Autodesk Inventor part; units mm, degrees
(part 2 of 2)
sketch "Sketch19" plane through (0, 0, 0.5) normal (0, 0, 1) x (1, 0, 0)
  circle A0 centre (5.5, -12.3356) radius 0.0625 projected
  line L0 (5.5548, -12.3056) -> (5.7, -12.3056)
  line L1 (5.5548, -12.3656) -> (5.7, -12.3656)
  line L2 (5.7, -12.2156) -> (5.7, -12.3056)
  line L3 (5.71, -12.2056) -> (5.79, -12.2056)
  line L4 (5.8, -12.2156) -> (5.8, -12.2256)
  arc A1 (5.71, -12.2056) -> (5.7, -12.2156) centre (5.71, -12.2156) ccw
  arc A2 (5.8, -12.2156) -> (5.79, -12.2056) centre (5.79, -12.2156) ccw
  line L5 (5.7, -12.4556) -> (5.7, -12.3656)
  line L6 (5.71, -12.4656) -> (5.79, -12.4656)
  line L7 (5.8, -12.4556) -> (5.8, -12.4456)
  arc A3 (5.7, -12.4556) -> (5.71, -12.4656) centre (5.71, -12.4556) ccw
  arc A4 (5.79, -12.4656) -> (5.8, -12.4556) centre (5.79, -12.4556) ccw
  circle A5 centre (7.5, -12.3356) radius 0.0625 projected
  line L8 (7.4452, -12.3056) -> (7.3, -12.3056)
  line L9 (7.4452, -12.3656) -> (7.3, -12.3656)
  line L10 (7.3, -12.2156) -> (7.3, -12.3056)
  line L11 (7.29, -12.2056) -> (7.21, -12.2056)
  line L12 (7.2, -12.2156) -> (7.2, -12.2256)
  arc A6 (7.3, -12.2156) -> (7.29, -12.2056) centre (7.29, -12.2156) ccw
  arc A7 (7.21, -12.2056) -> (7.2, -12.2156) centre (7.21, -12.2156) ccw
  arc A8 (7.29, -12.4656) -> (7.3, -12.4556) centre (7.29, -12.4556) ccw
  line L13 (7.3, -12.4556) -> (7.3, -12.3656)
  line L14 (7.29, -12.4656) -> (7.21, -12.4656)
  arc A9 (7.2, -12.4556) -> (7.21, -12.4656) centre (7.21, -12.4556) ccw
  line L15 (7.2, -12.4556) -> (7.2, -12.4456)
  line L16 (5.8, -12.4456) -> (7.2, -12.4456)
  line L17 (5.8, -12.2256) -> (7.2, -12.2256)
  line L18 (5.5548, -10.3056) -> (5.7, -10.3056)
  line L19 (5.5548, -10.3656) -> (5.7, -10.3656)
  line L20 (5.7, -10.2156) -> (5.7, -10.3056)
  line L21 (5.71, -10.2056) -> (5.79, -10.2056)
  line L22 (5.8, -10.2156) -> (5.8, -10.2256)
  arc A10 (5.71, -10.2056) -> (5.7, -10.2156) centre (5.71, -10.2156) ccw
  arc A11 (5.8, -10.2156) -> (5.79, -10.2056) centre (5.79, -10.2156) ccw
  arc A12 (5.7, -10.4556) -> (5.71, -10.4656) centre (5.71, -10.4556) ccw
  line L23 (5.7, -10.4556) -> (5.7, -10.3656)
  line L24 (5.71, -10.4656) -> (5.79, -10.4656)
  arc A13 (5.79, -10.4656) -> (5.8, -10.4556) centre (5.79, -10.4556) ccw
  line L25 (5.8, -10.4556) -> (5.8, -10.4456)
  line L26 (7.4452, -10.3056) -> (7.3, -10.3056)
  line L27 (7.4452, -10.3656) -> (7.3, -10.3656)
  line L28 (7.3, -10.4556) -> (7.3, -10.3656)
  arc A14 (7.29, -10.4656) -> (7.3, -10.4556) centre (7.29, -10.4556) ccw
  line L29 (7.29, -10.4656) -> (7.21, -10.4656)
  arc A15 (7.2, -10.4556) -> (7.21, -10.4656) centre (7.21, -10.4556) ccw
  line L30 (7.2, -10.2156) -> (7.2, -10.2256)
  line L31 (7.29, -10.2056) -> (7.21, -10.2056)
  line L32 (7.3, -10.2156) -> (7.3, -10.3056)
  arc A16 (7.3, -10.2156) -> (7.29, -10.2056) centre (7.29, -10.2156) ccw
  arc A17 (7.21, -10.2056) -> (7.2, -10.2156) centre (7.21, -10.2156) ccw
  line L33 (7.2, -10.4556) -> (7.2, -10.4456)
  line L34 (5.8, -10.4456) -> (7.2, -10.4456)
  line L35 (5.8, -10.2256) -> (7.2, -10.2256)
  line L36 (5.5548, -9.6806) -> (5.7, -9.6806)
  line L37 (5.5548, -9.7406) -> (5.7, -9.7406)
  line L38 (5.7, -9.5906) -> (5.7, -9.6806)
  line L39 (5.71, -9.5806) -> (5.79, -9.5806)
  line L40 (5.8, -9.5906) -> (5.8, -9.6006)
  arc A18 (5.71, -9.5806) -> (5.7, -9.5906) centre (5.71, -9.5906) ccw
  arc A19 (5.8, -9.5906) -> (5.79, -9.5806) centre (5.79, -9.5906) ccw
  arc A20 (5.7, -9.8306) -> (5.71, -9.8406) centre (5.71, -9.8306) ccw
  line L41 (5.7, -9.8306) -> (5.7, -9.7406)
  line L42 (5.71, -9.8406) -> (5.79, -9.8406)
  arc A21 (5.79, -9.8406) -> (5.8, -9.8306) centre (5.79, -9.8306) ccw
  line L43 (5.8, -9.8306) -> (5.8, -9.8206)
  line L44 (7.4452, -9.6806) -> (7.3, -9.6806)
  line L45 (7.4452, -9.7406) -> (7.3, -9.7406)
  line L46 (7.3, -9.8306) -> (7.3, -9.7406)
  arc A22 (7.29, -9.8406) -> (7.3, -9.8306) centre (7.29, -9.8306) ccw
  line L47 (7.29, -9.8406) -> (7.21, -9.8406)
  arc A23 (7.2, -9.8306) -> (7.21, -9.8406) centre (7.21, -9.8306) ccw
  line L48 (7.2, -9.5906) -> (7.2, -9.6006)
  line L49 (7.29, -9.5806) -> (7.21, -9.5806)
  line L50 (7.3, -9.5906) -> (7.3, -9.6806)
  arc A24 (7.3, -9.5906) -> (7.29, -9.5806) centre (7.29, -9.5906) ccw
  arc A25 (7.21, -9.5806) -> (7.2, -9.5906) centre (7.21, -9.5906) ccw
  line L51 (7.2, -9.8306) -> (7.2, -9.8206)
  line L52 (5.8, -9.8206) -> (7.2, -9.8206)
  line L53 (5.8, -9.6006) -> (7.2, -9.6006)
  line L54 (5.5548, -9.0556) -> (5.7, -9.0556)
  line L55 (5.5548, -9.1156) -> (5.7, -9.1156)
  line L56 (5.7, -8.9656) -> (5.7, -9.0556)
  line L57 (5.71, -8.9556) -> (5.79, -8.9556)
  line L58 (5.8, -8.9656) -> (5.8, -8.9756)
  arc A26 (5.71, -8.9556) -> (5.7, -8.9656) centre (5.71, -8.9656) ccw
  arc A27 (5.8, -8.9656) -> (5.79, -8.9556) centre (5.79, -8.9656) ccw
  arc A28 (5.7, -9.2056) -> (5.71, -9.2156) centre (5.71, -9.2056) ccw
  line L59 (5.7, -9.2056) -> (5.7, -9.1156)
  line L60 (5.71, -9.2156) -> (5.79, -9.2156)
  arc A29 (5.79, -9.2156) -> (5.8, -9.2056) centre (5.79, -9.2056) ccw
  line L61 (5.8, -9.2056) -> (5.8, -9.1956)
  line L62 (7.4452, -9.0556) -> (7.3, -9.0556)
  line L63 (7.4452, -9.1156) -> (7.3, -9.1156)
  line L64 (7.3, -9.2056) -> (7.3, -9.1156)
  arc A30 (7.29, -9.2156) -> (7.3, -9.2056) centre (7.29, -9.2056) ccw
  line L65 (7.29, -9.2156) -> (7.21, -9.2156)
  arc A31 (7.2, -9.2056) -> (7.21, -9.2156) centre (7.21, -9.2056) ccw
  line L66 (7.2, -8.9656) -> (7.2, -8.9756)
  line L67 (7.29, -8.9556) -> (7.21, -8.9556)
  line L68 (7.3, -8.9656) -> (7.3, -9.0556)
  arc A32 (7.3, -8.9656) -> (7.29, -8.9556) centre (7.29, -8.9656) ccw
  arc A33 (7.21, -8.9556) -> (7.2, -8.9656) centre (7.21, -8.9656) ccw
  line L69 (7.2, -9.2056) -> (7.2, -9.1956)
  line L70 (5.8, -9.1956) -> (7.2, -9.1956)
  line L71 (5.8, -8.9756) -> (7.2, -8.9756)
  line L72 (5.5548, -8.4306) -> (5.7, -8.4306)
  line L73 (5.5548, -8.4906) -> (5.7, -8.4906)
  line L74 (5.7, -8.3406) -> (5.7, -8.4306)
  line L75 (5.71, -8.3306) -> (5.79, -8.3306)
  line L76 (5.8, -8.3406) -> (5.8, -8.3506)
  arc A34 (5.71, -8.3306) -> (5.7, -8.3406) centre (5.71, -8.3406) ccw
  arc A35 (5.8, -8.3406) -> (5.79, -8.3306) centre (5.79, -8.3406) ccw
  arc A36 (5.7, -8.5806) -> (5.71, -8.5906) centre (5.71, -8.5806) ccw
  line L77 (5.7, -8.5806) -> (5.7, -8.4906)
  line L78 (5.71, -8.5906) -> (5.79, -8.5906)
  arc A37 (5.79, -8.5906) -> (5.8, -8.5806) centre (5.79, -8.5806) ccw
  line L79 (5.8, -8.5806) -> (5.8, -8.5706)
  line L80 (7.4452, -8.4306) -> (7.3, -8.4306)
  line L81 (7.4452, -8.4906) -> (7.3, -8.4906)
  line L82 (7.3, -8.5806) -> (7.3, -8.4906)
  arc A38 (7.29, -8.5906) -> (7.3, -8.5806) centre (7.29, -8.5806) ccw
  line L83 (7.29, -8.5906) -> (7.21, -8.5906)
  arc A39 (7.2, -8.5806) -> (7.21, -8.5906) centre (7.21, -8.5806) ccw
  line L84 (7.2, -8.3406) -> (7.2, -8.3506)
  line L85 (7.29, -8.3306) -> (7.21, -8.3306)
  line L86 (7.3, -8.3406) -> (7.3, -8.4306)
  arc A40 (7.3, -8.3406) -> (7.29, -8.3306) centre (7.29, -8.3406) ccw
  arc A41 (7.21, -8.3306) -> (7.2, -8.3406) centre (7.21, -8.3406) ccw
  line L87 (7.2, -8.5806) -> (7.2, -8.5706)
  line L88 (5.8, -8.5706) -> (7.2, -8.5706)
  line L89 (5.8, -8.3506) -> (7.2, -8.3506)
  line L90 (5.5548, -7.8056) -> (5.7, -7.8056)
  line L91 (5.5548, -7.8656) -> (5.7, -7.8656)
  line L92 (5.7, -7.7156) -> (5.7, -7.8056)
  line L93 (5.71, -7.7056) -> (5.79, -7.7056)
  line L94 (5.8, -7.7156) -> (5.8, -7.7256)
  arc A42 (5.71, -7.7056) -> (5.7, -7.7156) centre (5.71, -7.7156) ccw
  arc A43 (5.8, -7.7156) -> (5.79, -7.7056) centre (5.79, -7.7156) ccw
  arc A44 (5.7, -7.9556) -> (5.71, -7.9656) centre (5.71, -7.9556) ccw
  line L95 (5.7, -7.9556) -> (5.7, -7.8656)
  line L96 (5.71, -7.9656) -> (5.79, -7.9656)
  arc A45 (5.79, -7.9656) -> (5.8, -7.9556) centre (5.79, -7.9556) ccw
  line L97 (5.8, -7.9556) -> (5.8, -7.9456)
  line L98 (7.4452, -7.8056) -> (7.3, -7.8056)
  line L99 (7.4452, -7.8656) -> (7.3, -7.8656)
  line L100 (7.3, -7.9556) -> (7.3, -7.8656)
  arc A46 (7.29, -7.9656) -> (7.3, -7.9556) centre (7.29, -7.9556) ccw
  line L101 (7.29, -7.9656) -> (7.21, -7.9656)
  arc A47 (7.2, -7.9556) -> (7.21, -7.9656) centre (7.21, -7.9556) ccw
  line L102 (7.2, -7.7156) -> (7.2, -7.7256)
  line L103 (7.29, -7.7056) -> (7.21, -7.7056)
  line L104 (7.3, -7.7156) -> (7.3, -7.8056)
  arc A48 (7.3, -7.7156) -> (7.29, -7.7056) centre (7.29, -7.7156) ccw
  arc A49 (7.21, -7.7056) -> (7.2, -7.7156) centre (7.21, -7.7156) ccw
  line L105 (7.2, -7.9556) -> (7.2, -7.9456)
  line L106 (5.8, -7.9456) -> (7.2, -7.9456)
  line L107 (5.8, -7.7256) -> (7.2, -7.7256)
  line L108 (5.5548, -7.1806) -> (5.7, -7.1806)
  line L109 (5.5548, -7.2406) -> (5.7, -7.2406)
  line L110 (5.7, -7.0906) -> (5.7, -7.1806)
  line L111 (5.71, -7.0806) -> (5.79, -7.0806)
  line L112 (5.8, -7.0906) -> (5.8, -7.1006)
  arc A50 (5.71, -7.0806) -> (5.7, -7.0906) centre (5.71, -7.0906) ccw
  arc A51 (5.8, -7.0906) -> (5.79, -7.0806) centre (5.79, -7.0906) ccw
  arc A52 (5.7, -7.3306) -> (5.71, -7.3406) centre (5.71, -7.3306) ccw
  line L113 (5.7, -7.3306) -> (5.7, -7.2406)
  line L114 (5.71, -7.3406) -> (5.79, -7.3406)
  arc A53 (5.79, -7.3406) -> (5.8, -7.3306) centre (5.79, -7.3306) ccw
  line L115 (5.8, -7.3306) -> (5.8, -7.3206)
  line L116 (7.4452, -7.1806) -> (7.3, -7.1806)
  line L117 (7.4452, -7.2406) -> (7.3, -7.2406)
  line L118 (7.3, -7.3306) -> (7.3, -7.2406)
  arc A54 (7.29, -7.3406) -> (7.3, -7.3306) centre (7.29, -7.3306) ccw
  line L119 (7.29, -7.3406) -> (7.21, -7.3406)
  arc A55 (7.2, -7.3306) -> (7.21, -7.3406) centre (7.21, -7.3306) ccw
  line L120 (7.2, -7.0906) -> (7.2, -7.1006)
  line L121 (7.29, -7.0806) -> (7.21, -7.0806)
  line L122 (7.3, -7.0906) -> (7.3, -7.1806)
  arc A56 (7.3, -7.0906) -> (7.29, -7.0806) centre (7.29, -7.0906) ccw
  arc A57 (7.21, -7.0806) -> (7.2, -7.0906) centre (7.21, -7.0906) ccw
  line L123 (7.2, -7.3306) -> (7.2, -7.3206)
  line L124 (5.8, -7.3206) -> (7.2, -7.3206)
  line L125 (5.8, -7.1006) -> (7.2, -7.1006)
  line L126 (5.5548, -6.6806) -> (5.7, -6.6806)
  line L127 (5.5548, -6.7406) -> (5.7, -6.7406)
  line L128 (5.7, -6.5906) -> (5.7, -6.6806)
  line L129 (5.71, -6.5806) -> (5.79, -6.5806)
  line L130 (5.8, -6.5906) -> (5.8, -6.6006)
  arc A58 (5.71, -6.5806) -> (5.7, -6.5906) centre (5.71, -6.5906) ccw
  arc A59 (5.8, -6.5906) -> (5.79, -6.5806) centre (5.79, -6.5906) ccw
  arc A60 (5.7, -6.8306) -> (5.71, -6.8406) centre (5.71, -6.8306) ccw
  line L131 (5.7, -6.8306) -> (5.7, -6.7406)
  line L132 (5.71, -6.8406) -> (5.79, -6.8406)
  arc A61 (5.79, -6.8406) -> (5.8, -6.8306) centre (5.79, -6.8306) ccw
  line L133 (5.8, -6.8306) -> (5.8, -6.8206)
  line L134 (7.4452, -6.6806) -> (7.3, -6.6806)
  line L135 (7.4452, -6.7406) -> (7.3, -6.7406)
  line L136 (7.3, -6.8306) -> (7.3, -6.7406)
  arc A62 (7.29, -6.8406) -> (7.3, -6.8306) centre (7.29, -6.8306) ccw
  line L137 (7.29, -6.8406) -> (7.21, -6.8406)
  arc A63 (7.2, -6.8306) -> (7.21, -6.8406) centre (7.21, -6.8306) ccw
  line L138 (7.2, -6.5906) -> (7.2, -6.6006)
  line L139 (7.29, -6.5806) -> (7.21, -6.5806)
  line L140 (7.3, -6.5906) -> (7.3, -6.6806)
  arc A64 (7.3, -6.5906) -> (7.29, -6.5806) centre (7.29, -6.5906) ccw
  arc A65 (7.21, -6.5806) -> (7.2, -6.5906) centre (7.21, -6.5906) ccw
  line L141 (7.2, -6.8306) -> (7.2, -6.8206)
  line L142 (5.8, -6.8206) -> (7.2, -6.8206)
  line L143 (5.8, -6.6006) -> (7.2, -6.6006)
  circle A66 centre (5.5, -7.8356) radius 0.0625 projected
  circle A67 centre (5.5, -7.8356) radius 0.0625
  circle A68 centre (5.5, -7.2106) radius 0.0625 projected
  circle A69 centre (5.5, -7.2106) radius 0.0625
  circle A70 centre (5.5, -6.7106) radius 0.0625 projected
  circle A71 centre (5.5, -6.7106) radius 0.0625
  circle A72 centre (7.5, -7.2106) radius 0.0625 projected
  circle A73 centre (7.5, -7.2106) radius 0.0625
  circle A74 centre (7.5, -6.7106) radius 0.0625 projected
  circle A75 centre (7.5, -6.7106) radius 0.0625
  circle A76 centre (7.5, -7.8356) radius 0.0625 projected
  circle A77 centre (7.5, -7.8356) radius 0.0625
  circle A78 centre (7.5, -8.4606) radius 0.0625 projected
  circle A79 centre (7.5, -8.4606) radius 0.0625
  circle A80 centre (7.5, -9.0856) radius 0.0625 projected
  circle A81 centre (7.5, -9.0856) radius 0.0625
  circle A82 centre (5.5, -9.0856) radius 0.0625 projected
  circle A83 centre (5.5, -9.0856) radius 0.0625
  circle A84 centre (5.5, -8.4606) radius 0.0625 projected
  circle A85 centre (5.5, -8.4606) radius 0.0625
  circle A86 centre (5.5, -10.3356) radius 0.0625 projected
  circle A87 centre (5.5, -10.3356) radius 0.0625
  circle A88 centre (5.5, -9.7106) radius 0.0625 projected
  circle A89 centre (5.5, -9.7106) radius 0.0625
  circle A90 centre (7.5, -9.7106) radius 0.0625 projected
  circle A91 centre (7.5, -9.7106) radius 0.0625
  circle A92 centre (7.5, -10.3356) radius 0.0625 projected
  circle A93 centre (7.5, -10.3356) radius 0.0625
  point P0 (0, 0)
  constraints: 288 end point, 132 point on circle, 64 centre point, 32 tangent, 24 horizontal, 14 coincident, 8 equal radius, 8 parallel, 8 vertical, 42 other
extrude "Extrusion11" cut sketch "Sketch19" against normal blind 0.001 contours A0 L0 L2 A1 L3 A2 L4 L17 L12 A7 L11 A6 L10 L8 A5 L9 L13 A8 L14 A9 L15 L16 L7 A4 L6 A3 L5 L1 | L18 L20 A10 L21 A11 L22 L35 L30 A17 L31 A16 L32 L26 A92 L27 L28 A14 L29 A15 L33 L34 L25 A13 L24 A12 L23 L19 A86 | L36 L38 A18 L39 A19 L40 L53 L48 A25 L49 A24 L50 L44 A90 L45 L46 A22 L47 A23 L51 L52 L43 A21 L42 A20 L41 L37 A88 | L54 L56 A26 L57 A27 L58 L71 L66 A33 L67 A32 L68 L62 A80 L63 L64 A30 L65 A31 L69 L70 L61 A29 L60 A28 L59 L55 A82 | L72 L74 A34 L75 A35 L76 L89 L84 A41 L85 A40 L86 L80 A78 L81 L82 A38 L83 A39 L87 L88 L79 A37 L78 A36 L77 L73 A84 | L90 L92 A42 L93 A43 L94 L107 L102 A49 L103 A48 L104 L98 A76 L99 L100 A46 L101 A47 L105 L106 L97 A45 L96 A44 L95 L91 A66 | L108 L110 A50 L111 A51 L112 L125 L120 A57 L121 A56 L122 L116 A72 L117 L118 A54 L119 A55 L123 L124 L115 A53 L114 A52 L113 L109 A68 | L126 L128 A58 L129 A59 L130 L143 L138 A65 L139 A64 L140 L134 A74 L135 L136 A62 L137 A63 L141 L142 L133 A61 L132 A60 L131 L127 A70
sketch "Sketch20" plane through (0, 0, 0.5) normal (0, 0, 1) x (1, 0, 0)
  line L0 (9.2529, -6.0349) -> (9.353, -6.0349) construction
  line L1 (9.353, -6.0349) -> (9.353, -6.1134) construction
  line L2 (9.353, -6.1134) -> (9.2529, -6.1134) construction
  line L3 (9.2529, -6.1134) -> (9.2529, -6.0349) construction
  point P0 (0, 0)
  constraints: 2 other
sketch "Sketch21" plane through (0, 0, 0.5) normal (0, 0, 1) x (1, 0, 0)
  line L0 (2.475, -6) -> (2.475, -5.85)
  line L1 (2.475, -5.85) -> (2.775, -5.85)
  line L2 (2.775, -5.85) -> (2.775, -12.35)
  line L3 (2.775, -12.35) -> (2.475, -12.35)
  line L4 (2.475, -12.35) -> (2.475, -6)
  line L5 (6.4126, -6.6715) -> (6.6377, -6.6715) construction
  line L6 (6.6377, -6.6715) -> (6.6377, -6.7316) construction
  line L7 (6.6377, -6.7316) -> (6.4126, -6.7316) construction
  line L8 (6.4126, -6.7316) -> (6.4126, -6.6715) construction
  line L9 (6.4225, -7.1608) -> (6.6476, -7.1608) construction
  line L10 (6.6476, -7.1608) -> (6.6476, -7.221) construction
  line L11 (6.6476, -7.221) -> (6.4225, -7.221) construction
  line L12 (6.4225, -7.221) -> (6.4225, -7.1608) construction
  line L13 (6.4217, -7.788) -> (6.6468, -7.788) construction
  line L14 (6.6468, -7.788) -> (6.6468, -7.8482) construction
  line L15 (6.6468, -7.8482) -> (6.4217, -7.8482) construction
  line L16 (6.4217, -7.8482) -> (6.4217, -7.788) construction
  line L17 (3.1, -6) -> (3.1, -5.85)
  line L18 (3.725, -6) -> (3.725, -5.85)
  line L19 (4.35, -6) -> (4.35, -5.85)
  line L20 (3.1, -5.85) -> (3.4, -5.85)
  line L21 (3.4, -5.85) -> (3.4, -12.35)
  line L22 (3.4, -12.35) -> (3.1, -12.35)
  line L23 (3.1, -12.35) -> (3.1, -6)
  line L24 (3.725, -5.85) -> (4.025, -5.85)
  line L25 (4.025, -5.85) -> (4.025, -12.35)
  line L26 (4.025, -12.35) -> (3.725, -12.35)
  line L27 (3.725, -12.35) -> (3.725, -6)
  line L28 (4.35, -5.85) -> (4.65, -5.85)
  line L29 (4.65, -5.85) -> (4.65, -12.35)
  line L30 (4.65, -12.35) -> (4.35, -12.35)
  line L31 (4.35, -12.35) -> (4.35, -6)
  line L32 (6.4642, -8.4748) -> (6.4642, -8.4147) construction
  line L33 (6.4642, -8.4147) -> (6.6262, -8.4147) construction
  line L34 (6.6262, -8.4147) -> (6.6262, -8.4748) construction
  line L35 (6.6262, -8.4748) -> (6.4642, -8.4748) construction
  line L36 (6.4337, -9.0961) -> (6.4337, -9.036) construction
  line L37 (6.4337, -9.036) -> (6.6588, -9.036) construction
  line L38 (6.6588, -9.036) -> (6.6588, -9.0961) construction
  line L39 (6.6588, -9.0961) -> (6.4337, -9.0961) construction
  line L40 (6.4323, -9.7147) -> (6.4323, -9.6546) construction
  line L41 (6.4323, -9.6546) -> (6.6574, -9.6546) construction
  line L42 (6.6574, -9.6546) -> (6.6574, -9.7147) construction
  line L43 (6.6574, -9.7147) -> (6.4323, -9.7147) construction
  line L44 (6.4255, -10.3617) -> (6.4255, -10.3016) construction
  line L45 (6.4255, -10.3016) -> (6.6506, -10.3016) construction
  line L46 (6.6506, -10.3016) -> (6.6506, -10.3617) construction
  line L47 (6.6506, -10.3617) -> (6.4255, -10.3617) construction
  line L48 (6.4342, -12.383) -> (6.4342, -12.2817) construction
  line L49 (6.4342, -12.2817) -> (6.6593, -12.2817) construction
  line L50 (6.6593, -12.2817) -> (6.6593, -12.383) construction
  line L51 (6.6593, -12.383) -> (6.4342, -12.383) construction
  line L52 (5, -7) -> (4.35, -7)
  line L53 (4.35, -8.6523) -> (5.1177, -8.6523)
  line L54 (5.1177, -8.6523) -> (5.1177, -7)
  line L55 (5, -7) -> (5.1177, -7)
  line L56 (9.39, -10.3668) -> (9.39, -8.5018)
  line L57 (8.79, -8.5018) -> (8.79, -10.3668)
  line L58 (8.79, -9.4343) -> (8.79, -9.2843)
  line L59 (8.79, -9.2843) -> (8.89, -9.2843)
  line L60 (8.89, -9.2843) -> (8.89, -9.5843)
  line L61 (8.89, -9.5843) -> (8.79, -9.5843)
  line L62 (9.69, -9.4343) -> (9.69, -9.1843)
  line L63 (9.69, -9.1843) -> (9.39, -9.1843)
  line L64 (9.69, -9.4343) -> (9.69, -9.6843)
  line L65 (9.69, -9.6843) -> (9.39, -9.6843)
  line L66 (8.79, -8.5018) -> (9.39, -8.5018)
  line L67 (8.79, -10.3668) -> (9.39, -10.3668)
  line L68 (9.29, -9.4343) -> (9.29, -9.0843)
  line L69 (9.29, -9.0843) -> (9.39, -9.0843)
  line L70 (9.29, -9.4343) -> (9.29, -9.7843)
  line L71 (9.29, -9.7843) -> (9.39, -9.7843)
  point P0 (0, 0)
  constraints: 80 end point, 13 perpendicular, 9 point on line, 6 vertical, 4 horizontal, 1 midpoint, 16 other
sketch "Sketch22" plane through (0, 0, 0) normal (0, 0, -1) x (-1, 0, 0)
  circle A0 centre (-9.0887, -11.003) radius 0.1 projected
  line L0 (-9.3887, -11.003) -> (-9.3887, -10.703)
  circle A1 centre (-8.6887, -11.003) radius 0.1 projected
  line L1 (-8.3887, -11.003) -> (-8.3887, -10.703)
  line L2 (-8.3887, -10.703) -> (-9.3887, -10.703)
  circle A2 centre (-8.8887, -12.3316) radius 0.1 projected
  line L3 (-9.3887, -11.003) -> (-9.3887, -12.6316)
  line L4 (-9.3887, -12.6316) -> (-8.3887, -12.6316)
  line L5 (-8.3887, -12.6316) -> (-8.3887, -11.003)
  circle A3 centre (-8.2121, -3.39) radius 0.1 projected
  line L6 (-7.9121, -3.39) -> (-7.9121, -3.69)
  circle A4 centre (-8.4104, -2.44) radius 0.1 projected
  line L7 (-8.4104, -2.14) -> (-7.9121, -2.14)
  circle A5 centre (-8.6121, -3.3893) radius 0.1 projected
  line L8 (-8.9121, -3.3893) -> (-8.9121, -3.6893)
  line L9 (-7.9121, -3.69) -> (-8.9121, -3.6893)
  line L10 (-8.9121, -3.3893) -> (-8.9121, -2.4893)
  line L11 (-8.9121, -2.4893) -> (-8.9121, -2.14)
  line L12 (-8.4104, -2.14) -> (-8.9121, -2.14)
  line L13 (-7.9121, -3.39) -> (-7.9121, -2.14)
  point P0 (0, 0)
  constraints: 28 end point, 4 vertical, 2 perpendicular, 1 horizontal
extrude "Extrusion12" add sketch "Sketch22" along normal blind 0.001
sketch "Sketch23" plane through (0, 0, 0.5) normal (0, 0, 1) x (1, 0, 0)
  line L0 (6.4364, -6.8881) -> (6.5968, -6.8881) construction
  line L1 (6.5968, -6.8881) -> (6.5968, -6.992) construction
  line L2 (6.5968, -6.992) -> (6.4364, -6.992) construction
  line L3 (6.4364, -6.992) -> (6.4364, -6.8881) construction
  line L4 (6.4361, -7.4082) -> (6.5965, -7.4082) construction
  line L5 (6.5965, -7.4082) -> (6.5965, -7.5082) construction
  line L6 (6.5965, -7.5082) -> (6.4361, -7.5082) construction
  line L7 (6.4361, -7.5082) -> (6.4361, -7.4082) construction
  line L8 (6.4442, -8.0322) -> (6.6046, -8.0322) construction
  line L9 (6.6046, -8.0322) -> (6.6046, -8.1367) construction
  line L10 (6.6046, -8.1367) -> (6.4442, -8.1367) construction
  line L11 (6.4442, -8.1367) -> (6.4442, -8.0322) construction
  line L12 (6.4449, -8.6472) -> (6.6053, -8.6472) construction
  line L13 (6.6053, -8.6472) -> (6.6053, -8.7472) construction
  line L14 (6.6053, -8.7472) -> (6.4449, -8.7472) construction
  line L15 (6.4449, -8.7472) -> (6.4449, -8.6472) construction
  line L16 (6.4675, -9.2967) -> (6.6278, -9.2967) construction
  line L17 (6.6278, -9.2967) -> (6.6278, -9.3971) construction
  line L18 (6.6278, -9.3971) -> (6.4675, -9.3971) construction
  line L19 (6.4675, -9.3971) -> (6.4675, -9.2967) construction
  line L20 (6.4727, -9.9151) -> (6.6331, -9.9151) construction
  line L21 (6.6331, -9.9151) -> (6.6331, -10.0172) construction
  line L22 (6.6331, -10.0172) -> (6.4727, -10.0172) construction
  line L23 (6.4727, -10.0172) -> (6.4727, -9.9151) construction
  line L24 (6.4883, -10.5491) -> (6.6486, -10.5491) construction
  line L25 (6.6486, -10.5491) -> (6.6486, -10.6512) construction
  line L26 (6.6486, -10.6512) -> (6.4883, -10.6512) construction
  line L27 (6.4883, -10.6512) -> (6.4883, -10.5491) construction
  line L28 (5.5344, -10.7366) -> (6.1019, -10.7366) construction
  line L29 (6.1019, -10.7366) -> (6.1019, -11.0038) construction
  line L30 (6.1019, -11.0038) -> (5.5344, -11.0038) construction
  line L31 (5.5344, -11.0038) -> (5.5344, -10.7366) construction
  line L32 (5.6586, -11.1538) -> (5.8162, -11.1538) construction
  line L33 (5.8162, -11.1538) -> (5.8162, -11.2574) construction
  line L34 (5.8162, -11.2574) -> (5.6586, -11.2574) construction
  line L35 (5.6586, -11.2574) -> (5.6586, -11.1538) construction
  line L36 (6.912, -11.1463) -> (7.0674, -11.1463) construction
  line L37 (7.0674, -11.1463) -> (7.0674, -11.2466) construction
  line L38 (7.0674, -11.2466) -> (6.912, -11.2466) construction
  line L39 (6.912, -11.2466) -> (6.912, -11.1463) construction
  line L40 (6.4628, -12.5696) -> (6.6231, -12.5696) construction
  line L41 (6.6231, -12.5696) -> (6.6231, -12.6738) construction
  line L42 (6.6231, -12.6738) -> (6.4628, -12.6738) construction
  line L43 (6.4628, -12.6738) -> (6.4628, -12.5696) construction
  point P0 (0, 0)
  constraints: 22 other
sketch "Sketch24" plane through (0, 0, 0.5) normal (0, 0, 1) x (1, 0, 0)
  circle A0 centre (7.1, -11.7731) radius 0.0625 projected
  circle A1 centre (7.1, -11.7731) radius 0.0625
  circle A2 centre (5.5, -11.7731) radius 0.0625
  point P0 (0, 0)
  dimension "d499" = 0.125
  constraints: 2 centre point, 1 coincident
  measures "d499" diameter of A2
extrude "Extrusion13" cut sketch "Sketch24" against normal blind 10
sketch "Sketch25" plane through (0, 0, 0.5) normal (0, 0, 1) x (1, 0, 0)
  line L0 (5.6, -11.7431) -> (5.6, -11.6931)
  line L1 (5.6, -11.8031) -> (5.6, -11.8531)
  circle A0 centre (7.1, -11.7731) radius 0.0625 projected
  circle A1 centre (7.1, -11.7731) radius 0.0625
  line L2 (7.0452, -11.7431) -> (7, -11.7431)
  line L3 (7.0452, -11.8031) -> (7, -11.8031)
  line L4 (7, -11.7431) -> (7, -11.6931)
  line L5 (7, -11.8031) -> (7, -11.8531)
  line L6 (5.6, -11.6931) -> (7, -11.6931)
  line L7 (5.6, -11.8531) -> (7, -11.8531)
  line L8 (6.7486, -11.6931) -> (6.7486, -11.8531)
  line L9 (6.8097, -11.6931) -> (6.8097, -11.8531)
  line L10 (5.6, -11.8031) -> (5.5548, -11.8031)
  circle A2 centre (5.5, -11.7731) radius 0.0625
  line L11 (5.6, -11.7431) -> (5.5548, -11.7431)
  point P0 (0, 0)
  constraints: 24 end point, 4 horizontal, 4 point on circle, 4 point on line, 2 centre point, 2 perpendicular, 2 vertical, 1 coincident
extrude "Extrusion14" cut sketch "Sketch25" against normal blind 0.001 contours L0 L6 L8 L7 L1 L10 A2 L11 | L6 L9 L7 L8 | L6 L4 L2 A0 L3 L5 L7 L9
sketch "Sketch26" plane through (0, 0, 0.5) normal (0, 0, 1) x (1, 0, 0)
  line L0 (6.447, -11.9017) -> (6.6153, -11.9017) construction
  line L1 (6.6153, -11.9017) -> (6.6153, -12.002) construction
  line L2 (6.6153, -12.002) -> (6.447, -12.002) construction
  line L3 (6.447, -12.002) -> (6.447, -11.9017) construction
  point P0 (0, 0)
  constraints: 2 other
body "Solid1"
